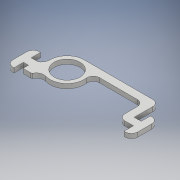
# Autodesk Inventor part: waterbottle_holder
Saved by Autodesk Inventor 2017.2 (Build 212233000, 233)
## iProperties
Created: 2017-07-16
Part Number: waterbottle_holder
Material: Generic
Document SubType Name: Modeling
Designer: Nic
Density: 1 g/cm^3
Appearance: Default
Author: Nic
Autodesk Inventor part; units mm, degrees
ref_plane "YZ Plane" through (0, 0, 0) normal (1, 0, 0) x (0, 1, 0)
ref_plane "XZ Plane" through (0, 0, 0) normal (0, 1, 0) x (-1, 0, 0)
ref_plane "XY Plane" through (0, 0, 0) normal (0, 0, 1) x (1, 0, 0)
sketch "Sketch1" plane through (0, 0, 0) normal (0, 0, 1) x (1, 0, 0)
  circle A0 centre (0, 0) radius 16.75
  line L0 (0, 0) -> (-17.65, 0) construction
  line L1 (-15.7399, -5.7288) -> (0, 0) construction
  line L2 (-14.2048, -8.8761) -> (0, 0) construction
  line L3 (-46, -6) -> (-46, -24)
  line L4 (-36.3668, 2) -> (-36.3668, -10)
  line L5 (-36.3668, -10) -> (-27.3668, -10)
  line L6 (-36.3668, -20) -> (-29.8668, -20)
  line L7 (-36.3668, -20) -> (-36.3668, -32)
  line L8 (-17.5898, -16) -> (-17.5898, -16)
  arc A1 (-27.3668, -10) -> (-22, 0) centre (-34, 0) ccw
  line L9 (34.6332, -10.9067) -> (34.6332, 21.7526) construction
  line L10 (115.2665, -6) -> (115.2665, -24)
  arc A2 (105.6332, -32) -> (115.2665, -24) centre (107.128, -24) ccw
  line L11 (105.6332, 2) -> (105.6332, -10)
  line L12 (105.6332, -10) -> (96.6332, -10)
  line L13 (105.6332, -20) -> (99.1332, -20)
  line L14 (105.6332, -20) -> (105.6332, -32)
  line L15 (96.6332, -10) -> (96.6332, 14)
  line L16 (0, 22) -> (88.6332, 22)
  line L17 (99.1332, -20) -> (94.6332, -20)
  line L18 (86.6332, -12) -> (86.6332, 4)
  line L19 (78.6332, 12) -> (29.7321, 12)
  arc A3 (96.6332, 14) -> (88.6332, 22) centre (88.6332, 14) ccw
  arc A4 (86.6332, 4) -> (78.6332, 12) centre (78.6332, 4) ccw
  arc A5 (86.6332, -12) -> (94.6332, -20) centre (94.6332, -12) ccw
  arc A6 (-6.3721, -21.057) -> (21.8036, 2.9333) centre (0, 0) ccw
  arc A7 (0, 22) -> (-22, 0) centre (0, 0) ccw
  arc A8 (29.7321, 12) -> (21.8036, 2.9333) centre (29.7321, 4) ccw
  line L20 (-19.8668, -27) -> (-29.8668, -27)
  line L21 (-29.8668, -27) -> (-29.8668, -20)
  line L22 (-46, -15) -> (-35.8797, -15) construction
  arc A9 (-6.3721, -21.057) -> (-18.1004, -25.9381) centre (-9.2685, -30.6283) ccw
  arc A10 (-19.8668, -27) -> (-18.1004, -25.9381) centre (-19.8668, -25) ccw
  arc A11 (-46, -24) -> (-36.3668, -32) centre (-37.8615, -24) ccw
  arc A12 (-36.3668, 2) -> (-46, -6) centre (-37.8615, -6) ccw
  arc A13 (115.2665, -6) -> (105.6332, 2) centre (107.128, -6) ccw
  point P0 (18.4391, 12)
  point P1 (-18.5871, -27)
  dimension "d12" = 16.75
  dimension "d19" = 160
  dimension "d30" = 9
  dimension "d40" = 46
  dimension "d43" = 8
  dimension "d44" = 22
  dimension "d45" = 8
  dimension "d46" = 10
  dimension "d47" = 10
  dimension "d48" = 142
  dimension "d59" = 6.5
  dimension "d61" = 10
  dimension "d63" = 12
  dimension "d65" = 10
  dimension "d66" = 2
  dimension "d67" = 10
  dimension "d68" = 10
  dimension "d69" = 7
  dimension "d70" = 5
  dimension "d71" = 12
  dimension "d72" = 18
  constraints: 46 end point, 35 point on circle, 15 tangent, 14 centre point, 10 symmetric about line, 6 horizontal, 5 vertical, 4 perpendicular, 3 equal radius, 2 coincident, 2 point on line, 1 collinear, 1 horizontal alignment, 1 midpoint, 3 other
  measures "d12" radius of A0
  measures "d19" angle of L0 L1
  measures "d30" distance of L4.end L5.end
  measures "d40" distance from line of L3 point (0, 0)
  measures "d43" radius of A3
  measures "d44" radius of A7
  measures "d45" radius of A8
  measures "d46" distance between parallel lines of L16 L19
  measures "d47" distance between parallel lines of L15 L18
  measures "d48" distance between parallel lines of L11 L4
  measures "d59" distance of L6.start L6.end
  measures "d61" radius of A9
  measures "d63" radius of A1
  measures "d65" distance between parallel lines of L0 L5
  measures "d66" radius of A10
  measures "d67" distance from line of L21 A10.centre
  measures "d68" distance between parallel lines of L5 L6
  measures "d69" distance between parallel lines of L6 L20
  measures "d70" distance between parallel lines of L22 L6
  measures "d71" distance of L4.start L4.end
  measures "d72" distance of L3.start L3.end
extrude "Extrusion1" add sketch "Sketch1" along normal blind 5.85
body "Solid1"
